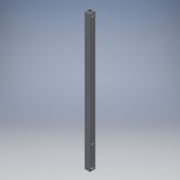
# Autodesk Inventor part: 26 inch 8th inch thick tube
Saved by Autodesk Inventor 2016 (Build 200138000, 138)
## iProperties
Created: 2016-02-05
Part Number: 26 inch 8th inch thick tube
Material: Generic
Document SubType Name: Modeling
Designer: gus
Density: 1 g/cm^3
Appearance: Default
Author: gus
Autodesk Inventor part; units mm, degrees
ref_plane "YZ Plane" through (0, 0, 0) normal (1, 0, 0) x (0, 1, 0)
ref_plane "XZ Plane" through (0, 0, 0) normal (0, 1, 0) x (-1, 0, 0)
ref_plane "XY Plane" through (0, 0, 0) normal (0, 0, 1) x (1, 0, 0)
sketch "Sketch1" plane through (0, 0, 0) normal (0, 1, 0) x (-1, 0, 0)
  line L0 (-1.9439, 0) -> (23.4561, 0)
  line L1 (23.4561, 0) -> (23.4561, 25.4)
  line L2 (23.4561, 25.4) -> (-1.9439, 25.4)
  line L3 (-1.9439, 25.4) -> (-1.9439, 0)
  line L4 (20.2811, 22.225) -> (1.2311, 22.225)
  line L5 (1.2311, 22.225) -> (1.2311, 3.175)
  line L6 (1.2311, 3.175) -> (20.2811, 3.175)
  line L7 (20.2811, 3.175) -> (20.2811, 22.225)
  point P0 (0, 0)
  dimension "d0" = 25.4
  dimension "d1" = 25.4
  dimension "d2" = 3.175
  dimension "d4" = 3.175
  dimension "d5" = 3.175
  dimension "d6" = 3.175
  constraints: 16 end point, 4 parallel, 2 horizontal, 2 perpendicular
  measures "d0" distance of L0.start L0.end
  measures "d1" distance of L2.end L0.start
  measures "d2" distance between parallel lines of L3 L5
  measures "d4" distance between parallel lines of L2 L4
  measures "d5" distance between parallel lines of L0 L6
  measures "d6" distance between parallel lines of L1 L7
extrude "Extrusion1" add sketch "Sketch1" along normal blind 660.4
sketch "Sketch2" plane through (1.9439, 0, 25.4) normal (1, 0, 0) x (0, 0, -1)
  circle A0 centre (12.7, 12.7) radius 6.35
  line L0 (25.4, 0) -> (25.4, 660.4) projected
  line L1 (0, 0) -> (25.4, 0) projected
  circle A1 centre (12.7, 647.7) radius 6.35
  line L2 (0, 660.4) -> (25.4, 660.4) projected
  dimension "d9" = 12.7
  dimension "d10" = 12.7
  dimension "d11" = 12.7
  dimension "d12" = 12.7
  dimension "d13" = 12.7
  dimension "d14" = 12.7
  constraints: 2 centre point
  measures "d9" diameter of A0
  measures "d10" distance from line of L0 A0.centre
  measures "d11" distance from line of L1 A0.centre
  measures "d12" diameter of A1
  measures "d13" distance from line of L0 A1.centre
  measures "d14" distance from line of L2 A1.centre
extrude "Extrusion2" cut sketch "Sketch2" against normal blind 660.4
sketch "Sketch3" plane through (1.9439, 0, 25.4) normal (1, 0, 0) x (0, 0, -1)
  circle A0 centre (12.7, 647.7) radius 6.35 projected
  circle A1 centre (12.7, 647.7) radius 6.35
  circle A2 centre (12.7, 12.7) radius 6.35
  circle A3 centre (12.7, 114.3) radius 6.35
  line L0 (0, 0) -> (25.4, 0) projected
  line L1 (25.4, 0) -> (25.4, 660.4) projected
  dimension "d17" = 12.7
  dimension "d18" = 12.7
  dimension "d19" = 12.7
  dimension "d20" = 12.7
  dimension "d21" = 101.6
  dimension "d22" = 12.7
  constraints: 3 centre point, 1 coincident
  measures "d17" diameter of A2
  measures "d18" distance from line of L0 A2.centre
  measures "d19" distance from line of L1 A2.centre
  measures "d20" diameter of A3
  measures "d21" distance of A2.centre A3.centre
  measures "d22" distance from line of L1 A3.centre
extrude "Extrusion3" cut sketch "Sketch3" against normal blind 660.4 contours A3
sketch "Sketch4" plane through (-23.4561, 0, 25.4) normal (0, 0, 1) x (1, 0, 0)
  point P0 (23.4561, 0)
sketch "Sketch5" plane through (1.9439, 0, 25.4) normal (1, 0, 0) x (0, 0, -1)
  circle A0 centre (12.7, 215.9) radius 6.35
  circle A1 centre (12.7, 114.3) radius 6.35 projected
  circle A2 centre (12.7, 114.3) radius 6.35
  line L0 (25.4, 0) -> (25.4, 660.4) projected
  dimension "d25" = 12.7
  dimension "d26" = 101.6
  dimension "d27" = 12.7
  constraints: 2 centre point, 1 coincident
  measures "d25" diameter of A0
  measures "d26" distance of A0.centre A2.centre
  measures "d27" distance from line of L0 A0.centre
extrude "Extrusion4" cut sketch "Sketch5" against normal blind 660.4 contours A0
body "Solid1"
